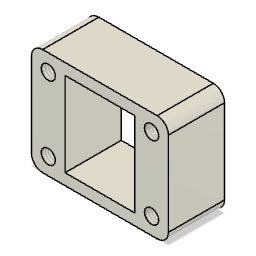
soporte_puenteH_v3 (Autodesk Fusion 360 design; units mm, degrees)
Autodesk Fusion 360 part; units mm, degrees
sketch "Sketch1" plane through (0, 0, 0) normal (0, 0, 1) x (1, 0, 0)
  line L0 (12.2, 9.5) -> (-12.2, 9.5)
  line L1 (-12.2, 9.5) -> (-12.2, -9.5)
  line L2 (-12.2, -9.5) -> (12.2, -9.5)
  line L3 (12.2, -9.5) -> (12.2, 9.5)
  line L4 (12.2, 9.5) -> (-12.2, -9.5) construction
  line L5 (-12.2, 9.5) -> (12.2, -9.5) construction
  line L6 (9.2, 6.5) -> (-9.2, 6.5) construction
  line L7 (-9.2, 6.5) -> (-9.2, -6.5) construction
  line L8 (-9.2, -6.5) -> (9.2, -6.5) construction
  line L9 (9.2, -6.5) -> (9.2, 6.5) construction
  line L10 (9.2, 6.5) -> (-9.2, -6.5) construction
  line L11 (-9.2, 6.5) -> (9.2, -6.5) construction
  circle A0 centre (9.2, 6.5) radius 1.5
  circle A1 centre (-9.2, -6.5) radius 1.5
  line L12 (0, 0) -> (9.2, 0) construction
  circle A2 centre (-9.2, 6.5) radius 1.5
  circle A3 centre (9.2, -6.5) radius 1.5
  line L13 (6.2, 7.5) -> (-6.2, 7.5)
  line L14 (-6.2, 7.5) -> (-6.2, -7.5)
  line L15 (-6.2, -7.5) -> (6.2, -7.5)
  line L16 (6.2, -7.5) -> (6.2, 7.5)
  line L17 (6.2, 7.5) -> (-6.2, -7.5) construction
  line L18 (-6.2, 7.5) -> (6.2, -7.5) construction
  dimension "d1" = 18.4
  dimension "d2" = 13
  dimension "d3" = 3
  dimension "d6" = 3
  dimension "d7" = 3
  dimension "d10" = 3
  dimension "d11" = 2
  constraint horizontal L0
  constraint perpendicular L0 L1
  constraint parallel L0 L2
  constraint parallel L1 L3
  constraint coincident L4 L12.start
  constraint coincident L5 L12.start
  constraint coincident L12.start origin
  constraint horizontal L6
  constraint perpendicular L6 L7
  constraint parallel L6 L8
  constraint parallel L7 L9
  constraint coincident L10 L12.start
  constraint coincident L11 L12.start
  constraint coincident L6.start L9.end
  constraint coincident L7.end L8.start
  constraint midpoint L9 L12.end
  constraint coincident L6.end L7.start
  constraint coincident L8.end L9.start
  constraint equal A0 A2
  constraint equal A0 A1
  constraint equal A0 A3
  constraint horizontal L13
  constraint perpendicular L13 L14
  constraint parallel L13 L15
  constraint parallel L14 L16
  constraint coincident L17 L12.start
  constraint coincident L18 L12.start
  measures "d1" distance of L6.start L6.end
  measures "d2" distance of L6.start L8.end
  measures "d3" diameter of A0
  measures "d6" distance of L3 L8.end
  measures "d7" distance of L2 L8.end
  measures "d10" distance of L6.start L16
  measures "d11" distance of L0 L13
extrude "Extrude1" add sketch "Sketch1" along normal blind 10
fillet "Fillet1" radius 2 4 edges at (12.2, -9.5, 5) (-12.2, -9.5, 5) (12.2, 9.5, 5) (-12.2, 9.5, 5)
thread "Thread1" "ISO Metric profile 3.0 M3x0.5 6H" major diameter 3.086 minor diameter 2.529 pitch 0.5 angle 60 resizes the face on face at (10.6981, 6.4252, 6.6667) on face at (-7.7019, 6.4252, 6.6667) on face at (10.6981, -6.5748, 6.6667) on face at (-7.7019, -6.5748, 6.6667)
